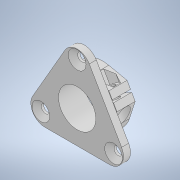
# Autodesk Inventor part: Motor Mount Insert
Saved by Autodesk Inventor 2022 (Build 260153000, 153)
## iProperties
Created: 2022-08-19
Part Number: Motor Mount Insert
Material: Generic
Document SubType Name: Modeling
Designer: Nick
Density: 1 g/cm^3
Appearance: Default
Mass: 4.06057 g
Surface Area: 35.3614 cm^2
Volume: 4.06057 cm^3
Author: Nick
Autodesk Inventor part; units mm, degrees
ref_plane "YZ Plane" through (0, 0, 0) normal (1, 0, 0) x (0, 1, 0)
ref_plane "XZ Plane" through (0, 0, 0) normal (0, 1, 0) x (-1, 0, 0)
ref_plane "XY Plane" through (0, 0, 0) normal (0, 0, 1) x (1, 0, 0)
sketch "Sketch1" plane through (0, 0, 0) normal (0, 0, 1) x (1, 0, 0)
  circle A0 centre (0, 16) radius 2
  circle A1 centre (-13.8564, -8) radius 2
  circle A2 centre (13.8564, -8) radius 2
  line L0 (0, 28) -> (24.2487, -14)
  line L1 (24.2487, -14) -> (-24.2487, -14)
  line L2 (-24.2487, -14) -> (0, 28)
  circle A3 centre (0, 0) radius 8
  line L3 (0, 16) -> (13.8564, -8) construction
  line L4 (13.8564, -8) -> (-13.8564, -8) construction
  line L5 (-13.8564, -8) -> (0, 16) construction
  dimension "d0" = 16
  dimension "d1" = 4
  dimension "d2" = 4
  dimension "d3" = 4
  dimension "d4" = 16
  dimension "d5" = 6
  constraints: 12 end point, 6 coincident, 4 centre point, 2 horizontal, 14 other
  measures "d0" diameter of A3
  measures "d1" diameter of A2
  measures "d2" diameter of A1
  measures "d3" diameter of A0
  measures "d4" distance of point (0, 0) A0.centre
  measures "d5" distance between parallel lines of L0 L3
extrude "Extrusion1" add sketch "Sketch1" along normal blind 3 contours A0 | A1 | A2 | L0 L1 L2
fillet "Fillet1" radius 6 3 edges at (0, 28, 1.5) (24.2487, -14, 1.5) (-24.2487, -14, 1.5)
sketch "Sketch2" plane through (0, 0, 0) normal (0, 0, -1) x (-1, 0, 0)
  circle A0 centre (0, 0) radius 8 projected
  arc A1 (13.8564, -14) -> (19.0526, -5) centre (13.8564, -8) ccw projected
  line L0 (5.1962, 19) -> (19.0526, -5) projected
  arc A2 (5.1962, 19) -> (-5.1962, 19) centre (0, 16) ccw projected
  line L1 (-19.0526, -5) -> (-5.1962, 19) projected
  arc A3 (-19.0526, -5) -> (-13.8564, -14) centre (-13.8564, -8) ccw projected
  line L2 (13.8564, -14) -> (-13.8564, -14) projected
  circle A4 centre (0, 0) radius 12
  line L3 (-10.6423, 5.567) -> (-10.1423, 6.433)
  line L4 (-10.1423, 6.433) -> (-6.6647, 4.4252)
  line L5 (-6.6647, 4.4252) -> (-7.1647, 3.5592)
  line L6 (-7.1647, 3.5592) -> (-10.6423, 5.567)
  line L7 (0, 0) -> (-6.9147, 3.9922) construction
  circle A5 centre (0, 0) radius 8 construction
  line L8 (-10.1423, 6.433) -> (-11.8744, 7.433)
  line L9 (-10.6423, 5.567) -> (-12.3744, 6.567)
  line L10 (-19.0526, -5) -> (-5.1962, 19) projected
  line L11 (-13.8744, 3.9689) -> (-11.427, -3.6639)
  line L12 (-10.3744, 10.0311) -> (-2.5404, 11.728)
  point P0 (-10.3744, 10.0311)
  point P1 (-12.3744, 6.567)
  point P2 (-13.8744, 3.9689)
  dimension "d9" = 4
  dimension "d10" = 1
  dimension "d11" = 3
  dimension "d12" = 3
  constraints: 18 end point, 5 perpendicular, 4 point on line, 3 point on circle, 3 tangent, 2 parallel, 1 centre point, 1 midpoint, 2 other
  measures "d10" distance between parallel lines of L6 L4
  measures "d11" distance of L9.end L11.start
  measures "d12" distance of L12.start L8.end
extrude "Extrusion2" add sketch "Sketch2" along normal blind 8 contours A0 L4 A4 L6 | L4 L8 L1 L12 A4 | A4 L11 L1 L9 L6 picked at (10.5558, -0.935)
sketch "Sketch3" plane through (6.6647, 4.4252, -8) normal (0.5, -0.8660254, 0) x (0.8660254, 0.5, 0)
  circle A0 centre (3.0078, 4) radius 1.5
  line L0 (0.2578, 5.5877) -> (3.0078, 7.1754)
  line L1 (3.0078, 7.1754) -> (5.7578, 5.5877)
  line L2 (5.7578, 5.5877) -> (5.7578, 2.4123)
  line L3 (5.7578, 2.4123) -> (3.0078, 0.8246)
  line L4 (3.0078, 0.8246) -> (0.2578, 2.4123)
  line L5 (0.2578, 2.4123) -> (0.2578, 5.5877)
  line L6 (6.0156, 8) -> (6.0156, 0) projected
  line L7 (6.0156, 0) -> (0, 0) projected
  point P0 (-7.9844, 8)
  point P1 (6.0156, 4)
  point P2 (3.0078, 0)
  dimension "d15" = 3
  dimension "d16" = 5.5
  constraints: 12 end point, 2 midpoint, 1 centre point, 1 coincident, 1 horizontal alignment, 1 vertical, 1 vertical alignment, 13 other
  measures "d15" diameter of A0
  measures "d16" distance between parallel lines of L2 L5
extrude "Extrusion3" cut sketch "Sketch3" against normal blind 8.75 contours A0 | L0 L1 L2 L3 L4 L5
extrude "Extrusion4" add sketch "Sketch3" against normal blind 3
sketch "Sketch4" plane through (12.3744, 6.567, 0) normal (-0.5, 0.8660254, 0) x (0.8660254, 0.5, 0)
  circle A0 centre (-3.0078, 4) radius 3
  circle A1 centre (-3.0078, 4) radius 1.5
  line L0 (-6.0156, 0) -> (-6.0156, 8) projected
  line L1 (-6.0156, 8) -> (0, 8) projected
  point P0 (-14, 0)
  point P1 (-6.0156, 4)
  point P2 (-3.0078, 8)
  dimension "d21" = 6
  dimension "d22" = 3
  constraints: 2 centre point, 2 midpoint, 1 coincident, 1 horizontal alignment, 1 vertical alignment
  measures "d21" diameter of A0
  measures "d22" diameter of A1
extrude "Extrusion5" cut sketch "Sketch4" against normal through all contours A0 | A1
extrude "Extrusion6" add sketch "Sketch4" against normal blind 3
sketch "Sketch5" plane through (0, 0, 0) normal (0, 0, -1) x (-1, 0, 0)
  line L0 (8.9761, 15.5471) -> (-8.9761, -15.5471)
  line L1 (-7.1647, 3.5592) -> (-12.3744, 6.567) projected
  line L2 (8.9761, 15.5471) -> (-21.6836, 15.1264)
  line L3 (-21.6836, 15.1264) -> (-8.9761, -15.5471)
  point P0 (0, 0)
  point P1 (0, 0)
  constraints: 6 end point, 1 coincident, 1 midpoint, 1 perpendicular
extrude "Extrusion7" cut sketch "Sketch5" along normal blind 0.2
chamfer "Chamfer1" distance 1 angle 45 1 edges at (9.9705, 1.715, -4)
sketch "Sketch6" plane through (0, 0, 3) normal (0, 0, 1) x (1, 0, 0)
  arc A0 (-19.0526, -5) -> (-13.8564, -14) centre (-13.8564, -8) ccw projected
  line L0 (-13.8564, -14) -> (13.8564, -14) projected
  arc A1 (13.8564, -14) -> (19.0526, -5) centre (13.8564, -8) ccw projected
  line L1 (19.0526, -5) -> (5.1962, 19) projected
  arc A2 (5.1962, 19) -> (-5.1962, 19) centre (0, 16) ccw projected
  line L2 (-5.1962, 19) -> (-19.0526, -5) projected
  circle A3 centre (0, 0) radius 8 projected
  line L3 (0, 0) -> (0, 18) construction
  line L4 (0, 0) -> (15.5885, -9) construction
  line L5 (0, 0) -> (-15.5885, -9) construction
  dimension "d32" = 2
  dimension "d33" = 2
  dimension "d34" = 2
  constraints: 6 end point, 3 point on line
  measures "d32" distance of A0.centre L5.end
  measures "d33" distance of L4.end A1.centre
  measures "d34" distance of A2.centre L3.end
hole "Hole1" at (0, 18, 3) at (15.5885, -9, 3) at (-15.5885, -9, 3) direction (0, 0, -1) diameter 3.6 end through all clearance for "Flat Head Machine Screw" size "M3" standard "Ansi Metric M Profile"
chamfer "Chamfer2" distance 2 angle 45 3 edges at (0, 19.8, 3) (-15.5885, -7.2, 3) (15.5885, -7.2, 3)
equation "\"d33\" = d32"
equation "\"d34\" = d32"
body "Solid1"
